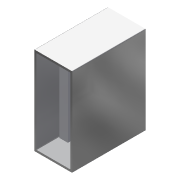
# Autodesk Inventor part: USBstick_halter
Saved by Autodesk Inventor 2017 (Build 210142000, 142)
## iProperties
Part Number: USBstick_halter
Material: Generisch
Document SubType Name: Modeling
Designer: ExCISS
Density: 1 g/cm^3
Appearance: Vorgabe
Author: ExCISS
Autodesk Inventor part; units mm, degrees
ref_plane "YZ Plane" through (0, 0, 0) normal (1, 0, 0) x (0, 1, 0)
ref_plane "XZ Plane" through (0, 0, 0) normal (0, 1, 0) x (-1, 0, 0)
ref_plane "XY Plane" through (0, 0, 0) normal (0, 0, 1) x (1, 0, 0)
sketch "Skizze1" plane through (0, 0, 0) normal (0, 0, 1) x (1, 0, 0)
  line L0 (-2.85, 5.47) -> (2.85, 5.47)
  line L1 (2.85, 5.47) -> (2.85, -5.47)
  line L2 (2.85, -5.47) -> (-2.85, -5.47)
  line L3 (-2.85, -5.47) -> (-2.85, 5.47)
  line L4 (-2.85, 5.47) -> (2.85, -5.47) construction
  point P0 (0, 0)
  point P1 (0, 0)
  dimension "d0" = 5.7
  dimension "d1" = 10.94
  constraints: 10 end point, 2 parallel, 1 coincident, 1 horizontal, 1 midpoint, 1 perpendicular
  measures "d0" distance of L1.end L2.end
  measures "d1" distance of L0.end L1.end
extrude "Extrusion1" add sketch "Skizze1" along normal blind 13.11
shell "Wandung1" thickness 0.31 removed faces 1 at (0.95, -5.47, 4.37)
fillet "Rundung1" radius 0.1 8 edges at (2.85, 0, 13.11) (-2.85, 0, 13.11) (2.85, 0, 0) (-2.85, 0, 0) (2.54, -0.155, 12.8) (-2.54, -0.155, 12.8) (-2.54, -0.155, 0.31) (2.54, -0.155, 0.31)
sketch "Skizze2" plane through (-2.44, 5.16, 12.8) normal (0, -1, 0) x (1, 0, 0)
  arc A0 (4.88, -12.49) -> (4.98, -12.39) centre (4.88, -12.39) ccw construction
  line L0 (4.88, -12.39) -> (2.3, -12.39) construction
  line L1 (2.3, -12.39) -> (2.3, -11.55) construction
  line L2 (2.3, -11.55) -> (4.88, -11.55) construction
  line L3 (4.88, -11.55) -> (4.88, -12.39) construction
  arc A1 (4.98, -0.1) -> (4.88, 0) centre (4.88, -0.1) ccw construction
  line L4 (4.88, -0.1) -> (2.3, -0.1) construction
  line L5 (2.3, -0.1) -> (2.3, -0.94) construction
  line L6 (2.3, -0.94) -> (4.88, -0.94) construction
  line L7 (4.88, -0.94) -> (4.88, -0.1) construction
  line L8 (-0.1, -12.39) -> (-0.1, -0.1) construction
  line L9 (-0.1, -6.245) -> (1.03, -6.245) construction
  line L10 (2.3, -0.94) -> (1.03, -0.94)
  line L11 (1.03, -0.94) -> (1.03, -11.55)
  line L12 (1.03, -11.55) -> (2.3, -11.55)
  line L13 (2.3, -11.55) -> (2.3, -0.94)
  point P0 (2.44, -12.8)
  dimension "d6" = 2.58
  dimension "d7" = 0.84
  dimension "d8" = 2.58
  dimension "d9" = 0.84
  dimension "d10" = 1.13
  constraints: 26 end point, 6 parallel, 4 horizontal, 3 perpendicular, 1 midpoint
  measures "d6" distance of L1.end L2.end
  measures "d7" distance of L0.end L1.end
  measures "d8" distance of L6.end L5.end
  measures "d9" distance of L5.end L4.end
  measures "d10" distance of L9.start L9.end
extrude "Extrusion2" add sketch "Skizze2" along normal blind 8.32
